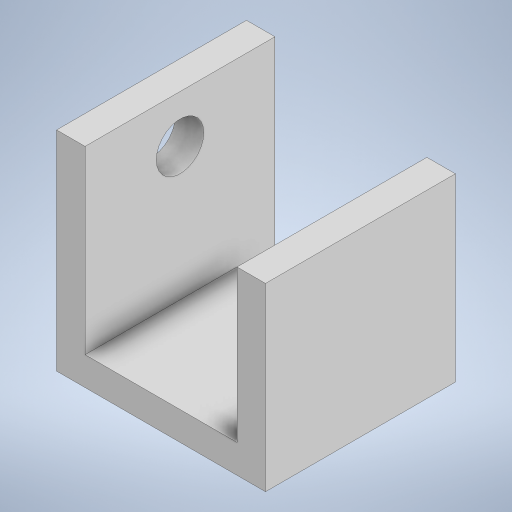
# Autodesk Inventor part: LED strip mount v01
Saved by Autodesk Inventor 2023 (Build 270158000, 158)
## iProperties
Created: 2024-06-26
Part Number: LED strip mount v01
Material: Generic
Document SubType Name: Modeling
Designer: Akramilab
Density: 1 g/cm^3
Appearance: Default
Author: Akramilab
Autodesk Inventor part; units mm, degrees
ref_plane "YZ Plane" through (0, 0, 0) normal (1, 0, 0) x (0, 1, 0)
ref_plane "XZ Plane" through (0, 0, 0) normal (0, 1, 0) x (-1, 0, 0)
ref_plane "XY Plane" through (0, 0, 0) normal (0, 0, 1) x (1, 0, 0)
sketch "Sketch1" plane through (0, 0, 0) normal (0, 0, 1) x (1, 0, 0)
  line L0 (0, 0) -> (22, 0)
  line L1 (22, 0) -> (22, -19)
  line L2 (22, -19) -> (0, -19)
  line L3 (0, -19) -> (0, 0)
  line L4 (3, 0) -> (19, 0)
  line L5 (19, 0) -> (19, -16)
  line L6 (19, -16) -> (3, -16)
  line L7 (3, -16) -> (3, 0)
  dimension "d0" = 22
  dimension "d1" = 19
  dimension "d2" = 3
  dimension "d3" = 3
  dimension "d4" = 3
  constraints: 16 end point, 4 parallel, 2 horizontal, 2 perpendicular, 1 point on line
  measures "d0" distance between parallel lines of L1 L3
  measures "d1" distance between parallel lines of L2 L0
  measures "d2" distance between parallel lines of L7 L3
  measures "d3" distance between parallel lines of L2 L6
  measures "d4" distance between parallel lines of L5 L1
extrude "Extrusion1" add sketch "Sketch1" along normal blind 20 contours L0 L7 L6 L5 L1 L2 L3
sketch "Sketch2" plane through (0, -19, 0) normal (-1, 0, 0) x (0, 0, 1)
  line L0 (0, 19) -> (20, 19) projected
  line L1 (0, 19) -> (20, 19)
  line L2 (20, 19) -> (20, 22)
  line L3 (20, 22) -> (0, 22)
  line L4 (0, 22) -> (0, 19)
  dimension "d7" = 3
  constraints: 8 end point, 2 parallel, 1 horizontal, 1 perpendicular
  measures "d7" distance of L2.end L1.end
extrude "Extrusion2" add sketch "Sketch2" against normal blind 3
sketch "Sketch3" plane through (0, -19, 0) normal (-1, 0, 0) x (0, 0, 1)
  line L0 (0, 22) -> (0, 0) projected
  line L1 (20, 22) -> (0, 22) projected
  circle A0 centre (10, 17) radius 2.5
  point P0 (0, 19)
  dimension "d10" = 10
  dimension "d11" = 5
  dimension "d12" = 5
  constraints: 1 centre point, 1 coincident
  measures "d10" distance from line of L0 point (10, 17)
  measures "d11" distance from line of point (10, 17) L1
  measures "d12" diameter of A0
extrude "Extrusion3" cut sketch "Sketch3" against normal blind 5
equation "\"d3\" = d2"
equation "\"d4\" = d2"
body "Solid1"
